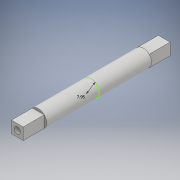
# Autodesk Inventor part: crankshaft_bearing_mounts
Saved by Autodesk Inventor 2018 (Build 220112000, 112)
## iProperties
Created: 2026-05-02
Part Number: crankshaft_bearing_mounts
Material: Generic
Document SubType Name: Modeling
Designer: neo
Density: 1 g/cm^3
Appearance: Default
Author: neo
Autodesk Inventor part; units mm, degrees
ref_plane "YZ Plane" through (0, 0, 0) normal (1, 0, 0) x (0, 1, 0)
ref_plane "XZ Plane" through (0, 0, 0) normal (0, 1, 0) x (-1, 0, 0)
ref_plane "XY Plane" through (0, 0, 0) normal (0, 0, 1) x (1, 0, 0)
sketch "Sketch1" plane through (0, 0, 0) normal (0, 1, 0) x (-1, 0, 0)
  line L0 (2.0677, 2.6131) -> (-3.5538, 2.6131)
  line L1 (-3.5538, 2.6131) -> (-3.5538, -3.0084)
  line L2 (-3.5538, -3.0084) -> (2.0677, -3.0084)
  line L3 (2.0677, -3.0084) -> (2.0677, 2.6131)
  circle A0 centre (-0.743, -0.1977) radius 3.975
  point P0 (0, 0)
  dimension "d0" = 7.95
  constraints: 8 end point, 3 point on circle, 2 parallel, 2 perpendicular, 1 centre point, 1 horizontal
  measures "d0" diameter of A0
extrude "Extrusion1" add sketch "Sketch1" along normal mid plane 50
extrude "Extrusion2" add sketch "Sketch1" along normal mid plane 70 contours L3 L2 L1 L0
hole "Hole1" at (0.743, -35, -0.1977) direction (0, 1, 0) diameter 3 end through all
body "Solid1"
